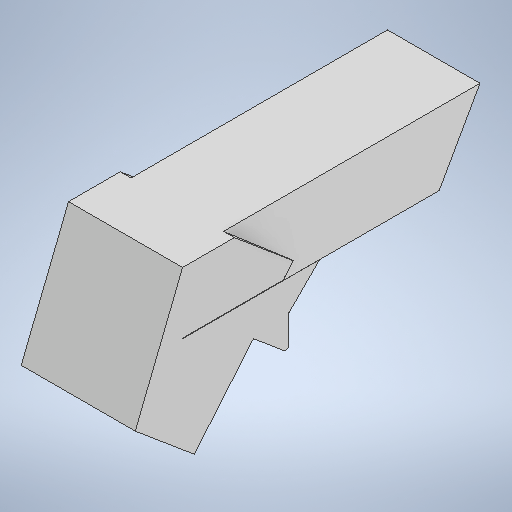
# Autodesk Inventor part: palitowantan
Saved by Autodesk Inventor 2025.1 (Build 291241020, 241B)
## iProperties
Created: 2024-11-26
Part Number: palitowantan
Material: Genérico
Document SubType Name: Modeling
Designer: ctamashiro
Density: 1 g/cm^3
Appearance: Valor por defecto
Author: ctamashiro
Autodesk Inventor part; units mm, degrees
ref_plane "YZ Plane" through (0, 0, 0) normal (1, 0, 0) x (0, 1, 0)
ref_plane "XZ Plane" through (0, 0, 0) normal (0, 1, 0) x (-1, 0, 0)
ref_plane "XY Plane" through (0, 0, 0) normal (0, 0, 1) x (1, 0, 0)
sketch "Boceto1" plane through (0, 0, 0) normal (0, 1, 0) x (-1, 0, 0)
  line L0 (-3, -10) -> (3, -10)
  line L1 (3, -10) -> (3, 10)
  line L2 (3, 10) -> (-3, 10)
  line L3 (-3, 10) -> (-3, -10)
  line L4 (-3, -10) -> (3, 10) construction
  line L5 (3, -10) -> (-3, 10) construction
  point P0 (0, 0)
  dimension "d0" = 6
  dimension "d1" = 20
  constraints: 12 end point, 2 midpoint, 2 parallel, 1 horizontal, 1 perpendicular
  measures "d0" distance of L2.end L1.end
  measures "d1" distance of L1.end L0.end
extrude "Extrusión1" add sketch "Boceto1" along normal blind 4
sketch "Boceto2" plane through (-3, 0, -10) normal (-1, 0, 0) x (0, 0, 1)
  line L0 (0, 0) -> (0, 4) projected
  line L1 (0, 4) -> (3.3564, 0)
  line L2 (0, 0) -> (20, 0) projected
  line L3 (0, 4) -> (5.2216, 4) construction
  line L4 (3.3564, 0) -> (0, 0)
  line L5 (0, 0) -> (0, 4)
  line L6 (20, 0) -> (16.6436, 4)
  line L7 (0, 4) -> (20, 4) projected
  line L8 (20, 0) -> (25.2216, 0) construction
  line L9 (16.6436, 4) -> (12.8134, 0.7861)
  line L10 (12.8134, 0.7861) -> (19.2413, -6.8744)
  line L11 (19.2413, -6.8744) -> (23.0715, -3.6604)
  line L12 (23.0715, -3.6604) -> (20, 0)
  line L13 (20, 4) -> (23.0715, -3.6604)
  line L14 (20, 4) -> (16.6436, 4)
  line L15 (13.473, 0) -> (15.4013, -2.2981)
  line L16 (15.4013, -2.2981) -> (13.1032, -4.2265)
  line L17 (13.1032, -4.2265) -> (13.1032, 0)
  point P0 (10, 0)
  point P1 (14.7285, 2.393)
  point P2 (14.8694, 0)
  point P3 (11.8766, 0)
  dimension "d9" = 50
  dimension "d10" = 130
  dimension "d11" = 90
  dimension "d12" = 10
  dimension "d15" = 5
  dimension "d16" = 3
  dimension "d17" = 3
  constraints: 30 end point, 6 point on line, 3 collinear, 2 equal length, 2 horizontal, 2 parallel, 2 perpendicular, 1 midpoint
  measures "d9" angle of L1 L3
  measures "d10" angle of L8 L6
  measures "d11" angle of L10 L9
  measures "d12" distance from line of L11 point (14.728, 2.393)
  measures "d15" distance between parallel lines of L10 L12
  measures "d16" distance of L15.start L15.end
  measures "d17" distance of L15.end L16.end
draft "Cara para el ángulo de desmoldeo1" angle 10 pull direction (0, 1, 0) faces at (3, 2.6667, 3.3333) fixed edges at (3, 4, 0)
mirror "Simetría1" about plane through (0, 0, 0) normal (1, 0, 0) of "Extrusión1", "Cara para el ángulo de desmoldeo1"
extrude "Extrusión2" cut sketch "Boceto2" along normal mid plane 20 contours L0 L1 L2
extrude "Extrusión3" add sketch "Boceto2" along normal blind 0.7 and the other way blind 6.7 contours L7 L13 L12 L6 | L6 L2 L10 L9 | L2 L10 L16 L17 | L12 L11 L10 L2
chamfer "Chaflán1" distance 2 angle 45 1 edges at (0, 0, 3.1032)
fillet "Empalme1" radius 0.2 1 edges at (0, -4.2265, 3.1032)
